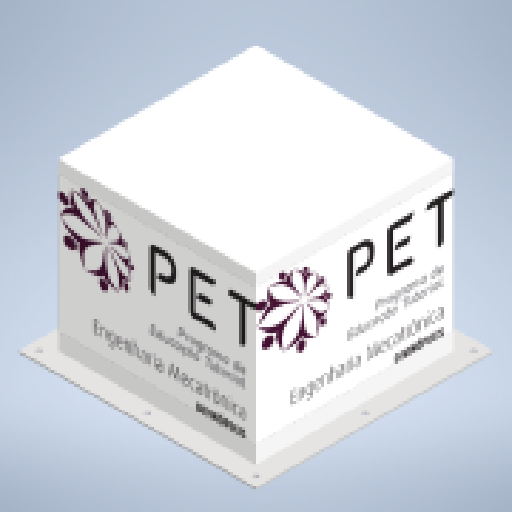
# Autodesk Inventor part: parte1
Saved by Autodesk Inventor 2023 (Build 270158000, 158)
## iProperties
Created: 2023-03-07
Part Number: parte1
Material: Generic
Document SubType Name: Modeling
Designer: klebe
Density: 1 g/cm^3
Appearance: Default
Author: klebe
Autodesk Inventor part; units mm, degrees
ref_plane "YZ Plane" through (0, 0, 0) normal (1, 0, 0) x (0, 1, 0)
ref_plane "XZ Plane" through (0, 0, 0) normal (0, 1, 0) x (-1, 0, 0)
ref_plane "XY Plane" through (0, 0, 0) normal (0, 0, 1) x (1, 0, 0)
sketch "Sketch1" plane through (0, 0, 0) normal (0, 1, 0) x (-1, 0, 0)
  line L0 (0, 0) -> (1000, 0)
  line L1 (1000, 0) -> (1000, 1000)
  line L2 (1000, 1000) -> (0, 1000)
  line L3 (0, 1000) -> (0, 0)
  line L4 (-100, 1100) -> (1100, 1100)
  line L5 (1100, 1100) -> (1100, -100)
  line L6 (1100, -100) -> (-100, -100)
  line L7 (-100, -100) -> (-100, 1100)
  dimension "d0" = 1000
  dimension "d1" = 1000
  dimension "d2" = 100
  constraints: 16 end point, 4 parallel, 2 perpendicular, 1 horizontal, 3 other
  measures "d0" distance of L2.end L1.end
  measures "d1" distance of L1.end L0.end
  measures "d2" distance between parallel lines of L2 L4
extrude "Extrusion1" add sketch "Sketch1" along normal blind 850 contours L3 L2 L1 L0
extrude "Extrusion2" add sketch "Sketch1" along normal blind 10
sketch "Sketch2" plane through (0, 10, 0) normal (0, 1, 0) x (1, 0, 0)
  line L0 (100, 100) -> (-1100, 100) projected
  line L1 (-1100, 100) -> (-1100, -1100) projected
  line L2 (-1100, -1100) -> (100, -1100) projected
  line L3 (100, -1100) -> (100, 100) projected
  line L4 (0, -1000) -> (0, 0) projected
  line L5 (-1000, -1000) -> (0, -1000) projected
  line L6 (-1000, 0) -> (-1000, -1000) projected
  line L7 (0, 0) -> (-1000, 0) projected
  line L8 (-1000, -1000) -> (-1050, -1000)
  line L9 (-1050, -1000) -> (-1050, -1050)
  line L10 (-1050, -1050) -> (50, -1050)
  line L11 (50, -1050) -> (50, 50)
  line L12 (50, 50) -> (-1050, 50)
  line L13 (-1050, 50) -> (-500, 50)
  line L14 (-500, 50) -> (-500, -1050)
  line L15 (50, 50) -> (50, -500)
  line L16 (50, -500) -> (-1000, -500)
  line L17 (-1000, -500) -> (-1050, -500)
  dimension "d7" = 50
  dimension "d8" = 50
  dimension "d9" = 1100
  dimension "d10" = 1100
  dimension "d11" = 550
  constraints: 20 end point, 5 perpendicular, 4 midpoint, 1 horizontal, 1 point on line
  measures "d7" distance of L5.start L8.end
  measures "d8" distance of L8.end L9.end
  measures "d9" distance of L9.end L10.end
  measures "d10" distance of L10.end L11.end
  measures "d11" distance of L12.end L13.end
hole "Hole1" at (-1050, 10, 1050) at (-500, 10, 1050) at (50, 10, 1050) at (50, 10, -50) at (-500, 10, -50) at (-1050, 10, -50) at (50, 10, 500) at (-1050, 10, 500) direction (0, -1, 0) diameter 25.4 end through all
sketch "Sketch3" plane through (0, 850, 1000) normal (1, 0, 0) x (0, 0, -1)
  line L0 (0, -59.4954) -> (1000, -59.4954) construction
  line L1 (1000, -59.4954) -> (1000, -749.3909) construction
  line L2 (1000, -749.3909) -> (0, -749.3909) construction
  line L3 (0, -749.3909) -> (0, -59.4954) construction
  point P0 (1000, -850)
  constraints: 2 other
decal "Decal1"
sketch "Sketch4" plane through (-1000, 850, 1000) normal (0, 0, 1) x (1, 0, 0)
  line L0 (0, -840) -> (0, 0) projected
  line L1 (0, -64.0631) -> (1000, -64.0631) construction
  line L2 (1000, -64.0631) -> (1000, -753.9585) construction
  line L3 (1000, -753.9585) -> (0, -753.9585) construction
  line L4 (0, -753.9585) -> (0, -64.0631) construction
  point P0 (1000, -850)
  constraints: 2 other
decal "Decal2"
sketch "Sketch5" plane through (-1000, 850, 0) normal (-1, 0, 0) x (0, 0, 1)
  line L0 (57.8435, -18.5187) -> (921.1484, -18.5187) construction
  line L1 (921.1484, -18.5187) -> (921.1484, -825.537) construction
  line L2 (921.1484, -825.537) -> (57.8435, -825.537) construction
  line L3 (57.8435, -825.537) -> (57.8435, -18.5187) construction
  point P0 (0, -850)
  constraints: 2 other
decal "Decal3"
sketch "Sketch6" plane through (0, 850, 0) normal (0, 0, -1) x (-1, 0, 0)
  line L0 (-2.3743, -103.2912) -> (997.1946, -103.2912) construction
  line L1 (997.1946, -103.2912) -> (997.1946, -725.2451) construction
  line L2 (997.1946, -725.2451) -> (-2.3743, -725.2451) construction
  line L3 (-2.3743, -725.2451) -> (-2.3743, -103.2912) construction
  point P0 (0, -850)
  constraints: 2 other
decal "Decal4"
sketch "Sketch7" plane through (0, 0, 0) normal (0, -1, 0) x (1, 0, 0)
  circle A0 centre (-1050, 500) radius 12.7 projected
  circle A1 centre (-500, 500) radius 5
  point P0 (0, 0)
  dimension "d73" = 10
  constraints: 1 centre point
  measures "d73" diameter of A1
extrude "Extrusion3" cut sketch "Sketch7" against normal blind 1 contours A1
body "Solid1"
